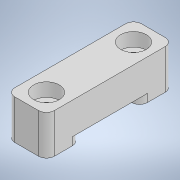
# Autodesk Inventor part: 32_Y-Motor_cable_holder_B
Saved by Autodesk Inventor 2022 (Build 260153000, 153)
## iProperties
Created: 2023-01-15
Part Number: 32_Y-Motor_cable_holder_B
Material: Generic
Document SubType Name: Modeling
Designer: Max
Density: 1 g/cm^3
Appearance: Default
Author: Max
Autodesk Inventor part; units mm, degrees
ref_plane "YZ Plane" through (0, 0, 0) normal (1, 0, 0) x (0, 1, 0)
ref_plane "XZ Plane" through (0, 0, 0) normal (0, 1, 0) x (-1, 0, 0)
ref_plane "XY Plane" through (0, 0, 0) normal (0, 0, 1) x (1, 0, 0)
sketch "Sketch1" plane through (0, 0, 0) normal (0, 1, 0) x (-1, 0, 0)
  line L0 (-5, 16) -> (5, 16)
  line L1 (5, 16) -> (5, -16)
  line L2 (5, -16) -> (-5, -16)
  line L3 (-5, -16) -> (-5, 16)
  line L4 (-5, 16) -> (5, -16) construction
  line L5 (5, 16) -> (-5, -16) construction
  point P0 (0, 0)
  dimension "d0" = 32
  dimension "d1" = 10
  constraints: 12 end point, 2 midpoint, 2 parallel, 1 horizontal, 1 perpendicular
  measures "d0" distance of L0.end L1.end
  measures "d1" distance between parallel lines of L3 L1
extrude "Extrusion1" add sketch "Sketch1" along normal blind 10
sketch "Sketch2" plane through (0, 10, 0) normal (0, 1, 0) x (1, 0, 0)
  line L0 (0, 22.4) -> (0, -22.4) projected
  line L1 (7, 0) -> (-7, 0) projected
  point P0 (0, 0)
  point P1 (0, -11)
  point P2 (0, 11)
  dimension "d4" = 22
  constraints: 1 point on line, 1 symmetric about line
  measures "d4" distance of point (0, 11) point (0, -11)
hole "Hole1" at (0, 10, 11) at (0, 10, -11) direction (0, -1, 0) diameter 3.4 depth 10 counterbore diameter 6.5 counterbore depth 3.4 clearance for "Socket Head Cap Screw ISO 4762" size "M3" standard "ISO"
fillet "Fillet1" radius 2 4 edges at (5, 5, 16) (-5, 5, 16) (5, 5, -16) (-5, 5, -16)
sketch "Sketch3" plane through (5, 0, 14) normal (1, 0, 0) x (0, 0, -1)
  line L0 (28, 0) -> (0, 0) projected
  line L1 (6.5, 0) -> (21.5, 0)
  line L2 (21.5, 0) -> (21.5, 2)
  line L3 (21.5, 2) -> (6.5, 2)
  line L4 (6.5, 2) -> (6.5, 0)
  line L5 (14, -2) -> (14, 12) projected
  point P0 (14, 0)
  dimension "d13" = 15
  dimension "d14" = 2
  constraints: 8 end point, 2 parallel, 1 horizontal, 1 perpendicular, 1 point on line, 1 other
  measures "d13" distance between parallel lines of L2 L4
  measures "d14" distance between parallel lines of L0 L3
extrude "Extrusion2" cut sketch "Sketch3" against normal through all
fillet "Fillet2" radius 2 4 edges at (5, 1, 7.5) (-5, 1, 7.5) (5, 1, -7.5) (-5, 1, -7.5)
body "Solid1"
